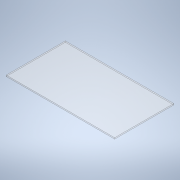
# Autodesk Inventor part: стекло
Saved by Autodesk Inventor 2022.4 (Build 264492010, 492A)
## iProperties
Created: 2023-02-20
Part Number: стекло
Material: Стекло, литое, прозрачное
Document SubType Name: Modeling
Designer: artyo
Density: 2.18 g/cm^3
Appearance: Бесцветный
Author: artyo
Autodesk Inventor part; units mm, degrees
ref_plane "YZ Plane" through (0, 0, 0) normal (1, 0, 0) x (0, 1, 0)
ref_plane "XZ Plane" through (0, 0, 0) normal (0, 1, 0) x (-1, 0, 0)
ref_plane "XY Plane" through (0, 0, 0) normal (0, 0, 1) x (1, 0, 0)
sketch "Эскиз1" plane through (0, 0, 0) normal (0, 1, 0) x (-1, 0, 0)
  line L0 (101.7322, 62.0786) -> (-74.2678, 62.0786)
  line L1 (-74.2678, 62.0786) -> (-74.2678, -33.9214)
  line L2 (-74.2678, -33.9214) -> (101.7322, -33.9214)
  line L3 (101.7322, -33.9214) -> (101.7322, 62.0786)
  line L4 (101.7322, 62.0786) -> (-74.2678, -33.9214) construction
  line L5 (-74.2678, 62.0786) -> (101.7322, -33.9214) construction
  point P0 (0, 0)
  point P1 (13.7322, 14.0786)
  dimension "d0" = 176
  dimension "d1" = 96
  constraints: 12 end point, 2 midpoint, 2 parallel, 1 horizontal, 1 perpendicular
  measures "d0" distance of L2.end L1.end
  measures "d1" distance of L1.end L0.end
extrude "Выдавливание1" add sketch "Эскиз1" along normal blind 2
